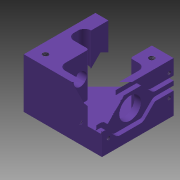
# Autodesk Inventor part: 13_1087_010
Saved by Autodesk Inventor 2014 SP1 (Build 180222100, 222)
## iProperties
Created: 2013-08-07
Part Number: 13_1087_010
Material: Allgemein
Document SubType Name: Modeling
Designer: vogel
Density: 1 g/cm^3
Appearance: Violett
Author: vogel
Autodesk Inventor part; units mm, degrees
note: some values were not read from the file. Chosen so that the rebuilt part matches the saved one: direction of "Bohrung2"; direction of "Bohrung3"; edges of "Rundung6".
ref_plane "YZ Plane" through (0, 0, 0) normal (1, 0, 0) x (0, 1, 0)
ref_plane "XZ Plane" through (0, 0, 0) normal (0, 1, 0) x (-1, 0, 0)
sketch "Skizze1" plane through (0, 0, 0) normal (0, 0, 1) x (1, 0, 0)
  line L0 (-25.2, 0) -> (25.2, 0) projected
  line L1 (0, -25.2) -> (0, 25.2) projected
  line L2 (-18, 18) -> (18, 18)
  line L3 (18, 18) -> (18, -18)
  line L4 (18, -18) -> (-18, -18)
  line L5 (-18, -18) -> (-18, 18)
  point P0 (0, 0)
  dimension "d0" = 36
  dimension "d1" = 36
  constraints: 8 end point, 2 parallel, 1 horizontal, 1 perpendicular, 2 other
  measures "d0" distance of L2.start L2.end
  measures "d1" distance of L4.end L2.start
extrude "Extrusion1" add sketch "Skizze1" along normal blind 23
shell "Hülle1" thickness 3 removed faces 1 at (6, -6, 23)
sketch "Skizze2" plane through (18, -18, 0) normal (1, 0, 0) x (0, 0, -1)
  line L0 (0, 36) -> (0, 0) projected
  line L1 (0, 36) -> (-23, 36) projected
  line L2 (0, 0) -> (-23, 0) projected
  line L3 (-13, 36) -> (-13, 0)
  line L4 (-3, 33) -> (-23, 33) projected
  point P0 (0, 18)
  point P1 (-13, 13)
  dimension "d5" = 13
  dimension "d30" = 20
  constraints: 3 point on line, 2 end point, 1 perpendicular
  measures "d5" distance between parallel lines of L3 L0
  measures "d30" distance from line of point (-13, 13) L4
sketch "Skizze3" plane through (-18, 18, 0) normal (0, 1, 0) x (1, 0, 0)
  line L0 (0, 0) -> (36, 0) projected
  line L1 (33, -3) -> (33, -23) projected
  line L2 (3, -3) -> (33, -3) projected
  line L3 (50, -7) -> (50, -17) projected
  point P0 (18, 0)
  point P1 (13, -13)
  dimension "d13" = 13
  dimension "d14" = 20
  measures "d13" distance from line of point (13, -13) L0
  measures "d14" distance from line of point (13, -13) L1
hole "Bohrung2" at (-5, 18, 13) direction (0, -1, 0) diameter 10 end up to surface
hole "Bohrung3" at (18, -5, 13) direction (-1, 0, 0) diameter 10 end up to surface
sketch "Skizze4" plane through (-15, 15, 3) normal (0, 0, 1) x (1, 0, 0)
  line L0 (0, -30) -> (0, 0) projected
  line L1 (30, -30) -> (0, -30) projected
  line L2 (0, -16) -> (10, -16)
  line L3 (10, -16) -> (10, -30)
  line L4 (10, -30) -> (0, -30)
  line L5 (0, -30) -> (0, -16)
  line L6 (30, 0) -> (23, 0)
  line L7 (23, 0) -> (23, -10)
  line L8 (23, -10) -> (30, -10)
  line L9 (30, -10) -> (30, 0)
  line L10 (0, 0) -> (30, 0) projected
  line L11 (3, 0) -> (0, 0)
  line L12 (0, 0) -> (0, -10)
  line L13 (0, -10) -> (3, -10)
  line L14 (3, -10) -> (3, 0)
  point P0 (15, -15)
  dimension "d31" = 14
  dimension "d32" = 10
  dimension "d40" = 10
  dimension "d41" = 7
  dimension "d46" = 3
  constraints: 24 end point, 6 parallel, 4 point on line, 3 horizontal, 3 perpendicular, 1 collinear
  measures "d31" distance of L4.end L2.start
  measures "d32" distance of L2.start L2.end
  measures "d40" distance between parallel lines of L6 L8
  measures "d41" distance of L7.end L8.end
  measures "d46" distance between parallel lines of L14 L12
extrude "Extrusion2" add sketch "Skizze4" along normal up to surface (20 mm away)
sketch "Skizze8" plane through (-15, 5, 3) normal (0, -1, 0) x (1, 0, 0)
  line L0 (3, 20) -> (0, 20) projected
  line L1 (0, 0) -> (0, 20) projected
  line L2 (3, 0) -> (0, 0) projected
  line L3 (3, 0) -> (3, 20) projected
  point P0 (15, -3)
extrude "Extrusion5" cut sketch "Skizze8" against normal blind 2
fillet "Rundung5" radius 1 2 edges at (-5, -1, 13) (8, 5, 13)
fillet "Rundung6" radius 3 5 edges at (-15, 7, 13) (-15, -1, 13) (-5, -15, 13) (15, -15, 13) (15, 5, 13)
sketch "Skizze9" plane through (18, -18, 0) normal (1, 0, 0) x (0, 0, -1)
  circle A0 centre (-13, 13) radius 5 projected
  point P0 (0, 18)
  constraints: 1 coincident
hole "Bohrung4" at (18, -5, 13) direction (-1, 0, 0) diameter 6 depth 27
sketch "Skizze10" plane through (0, 0, 23) normal (0, 0, 1) x (1, 0, 0)
  line L0 (-12, 15) -> (8, 15) projected
  line L1 (18, -18) -> (18, 18) projected
  line L2 (-18, 18) -> (18, 18)
  line L3 (18, 18) -> (18, 15)
  line L4 (18, 15) -> (-18, 15)
  line L5 (-18, 15) -> (-18, 18)
  point P0 (0, 0)
  constraints: 8 end point, 2 parallel, 1 collinear, 1 horizontal, 1 perpendicular, 1 point on line
extrude "Extrusion6" cut sketch "Skizze10" against normal through all
sketch "Skizze11" plane through (0, 0, 23) normal (0, 0, 1) x (1, 0, 0)
  line L0 (-18, -18) -> (18, -18) projected
  line L1 (-18, 15) -> (-18, -18) projected
  line L2 (18, 15) -> (-18, 15) projected
  line L3 (18, -18) -> (18, 15) projected
  circle A0 centre (-13, -13) radius 1.7 projected
  circle A1 centre (13, 10) radius 1.7 projected
  circle A2 centre (-13, -13) radius 1.7 projected
  point P0 (0, 0)
  point P1 (-13, -13)
  point P2 (13, 10)
hole "Bohrung5" at (-13, -13, 23) at (13, 10, 23) direction (0, 0, -1) diameter 2.459 depth 8 tip angle 118 thread size "M3x0.5" class "6H" standard "ISO Metric profile"
hole "Bohrung6" at (-5, -5, 13) direction (-1, 0, 0) diameter 4 depth 6 tip angle 118
sketch "Skizze12" plane through (-18, -18, 0) normal (0, -1, 0) x (1, 0, 0)
  line L0 (36, 0) -> (0, 0) projected
  line L1 (36, 0) -> (36, 23) projected
  line L2 (36, 9) -> (29.5, 9)
  line L3 (29.5, 9) -> (29.5, 17)
  line L4 (29.5, 17) -> (36, 17)
  line L5 (36, 17) -> (36, 9)
  circle A0 centre (22, 7) radius 2.2 projected
  circle A1 centre (22, 19) radius 2.2 projected
  circle A2 centre (4, 13) radius 2.2 projected
  circle A3 centre (33, 21) radius 1.2 projected
  circle A4 centre (3, 21) radius 1.2 projected
  circle A5 centre (3, 5) radius 1.2 projected
  circle A6 centre (33, 5) radius 1.2 projected
  circle A7 centre (8.5, 13) radius 0.9 projected
  circle A8 centre (17.5, 13) radius 0.9 projected
  circle A9 centre (13, 13) radius 3 projected
  line L6 (0, 0) -> (0, 26) projected
  line L7 (0, 0) -> (36, 0) projected
  line L8 (36, 0) -> (36, 26) projected
  line L9 (0, 26) -> (36, 26) projected
  point P0 (18, 0)
  dimension "d79" = 9
  dimension "d80" = 8
  dimension "d81" = 6.5
  dimension "d94" = 9
  constraints: 8 end point, 2 parallel, 1 horizontal, 1 perpendicular, 1 point on line
  measures "d79" distance between parallel lines of L2 L0
  measures "d80" distance of L2.end L3.end
  measures "d81" distance between parallel lines of L3 L1
  measures "d94" distance between parallel lines of L9 L4
extrude "Extrusion7" add sketch "Skizze12" along normal blind 8 contours L2 L3 L4 L1
sketch "Skizze14" plane through (18, -18, 0) normal (1, 0, 0) x (0, 0, -1)
  line L0 (0, 33) -> (-23, 33) projected
  line L1 (-23, 0) -> (-23, 33) projected
  line L2 (-9, -8) -> (-17, -8) projected
  line L3 (0, 0) -> (-9, 0) projected
  line L4 (0, 33) -> (0, 0) projected
  circle A0 centre (-13, 13) radius 5 projected
  line L5 (-11, -8) -> (-11, 1.1716)
  line L6 (-10.4142, 2.5858) -> (-6.0858, 6.9142)
  line L7 (-5.5, 8.3284) -> (-5.5, 17.6716)
  line L8 (-15, -8) -> (-15, 1.1716)
  line L9 (-15.5858, 2.5858) -> (-19.9142, 6.9142)
  line L10 (-20.5, 8.3284) -> (-20.5, 23.6063)
  line L11 (-13, 13) -> (-13, 24.4674)
  line L12 (-13, 24.4674) -> (-13, 13)
  line L13 (-10.2295, 13) -> (-13, 13)
  line L14 (-13, 13) -> (-13, -8)
  arc A1 (-10.4142, 2.5858) -> (-11, 1.1716) centre (-9, 1.1716) ccw
  arc A2 (-15, 1.1716) -> (-15.5858, 2.5858) centre (-17, 1.1716) ccw
  arc A3 (-20.5, 8.3284) -> (-19.9142, 6.9142) centre (-18.5, 8.3284) ccw
  arc A4 (-6.0858, 6.9142) -> (-5.5, 8.3284) centre (-7.5, 8.3284) ccw
  line L15 (-9, 0) -> (-9, -8) projected
  line L16 (-6.0858, 19.0858) -> (-10.4142, 23.4142)
  line L17 (-11, 24.8284) -> (-11, 33)
  arc A5 (-5.5, 17.6716) -> (-6.0858, 19.0858) centre (-7.5, 17.6716) ccw
  arc A6 (-11, 24.8284) -> (-10.4142, 23.4142) centre (-9, 24.8284) ccw
  point P0 (-17, 0)
  point P1 (0, 18)
  point P2 (-11, 2)
  point P3 (-5.5, 18.5)
  point P4 (-11, 24)
  dimension "d87" = 45
  dimension "d89" = 9
  dimension "d90" = 6
  dimension "d91" = 13
  dimension "d92" = 10
  dimension "d93" = 8
  dimension "d96" = 4
  dimension "d97" = 15
  dimension "d98" = 2
  dimension "d99" = 2
  dimension "d108" = 45
  dimension "d109" = 24
  dimension "d110" = 2
  dimension "d139" = 9
  constraints: 24 end point, 12 point on circle, 12 tangent, 9 point on line, 6 centre point, 6 parallel, 4 equal radius, 2 collinear, 2 perpendicular, 1 midpoint, 3 other
  measures "d87" angle of L3 L6
  measures "d89" distance of L3.start L3.end
  measures "d90" distance of point (-17, 0) L1.start
  measures "d91" distance between parallel lines of L4 L11
  measures "d92" distance between parallel lines of L1 L11
  measures "d93" distance of L2.start L2.end
  measures "d96" distance of L8.start L5.start
  measures "d97" distance between parallel lines of L7 L10
  measures "d98" distance from line of point (-11, 2) L3
  measures "d99" radius of A1
  measures "d108" angle of L16 L0
  measures "d109" distance from line of point (-11, 24) L3
  measures "d110" radius of A5
  measures "d139" distance from line of point (-11, 24) L0
sketch "Skizze15" plane through (-18, -26, 0) normal (0, -1, 0) x (1, 0, 0)
  line L0 (36, 9) -> (36, 17) projected
  line L1 (36, 10) -> (34, 10)
  line L2 (34, 10) -> (34, 12)
  line L3 (34, 12) -> (36, 12)
  line L4 (36, 12) -> (36, 10)
  line L5 (36, 14) -> (34, 14)
  line L6 (34, 14) -> (34, 16)
  line L7 (34, 16) -> (36, 16)
  line L8 (36, 16) -> (36, 14)
  line L9 (36, 15) -> (34, 15)
  line L10 (36, 11) -> (34.6551, 11)
  point P0 (18, 0)
  point P1 (36, 15)
  point P2 (36, 11)
  dimension "d100" = 2
  dimension "d101" = 2
  dimension "d102" = 2
  dimension "d103" = 2
  constraints: 20 end point, 4 parallel, 4 perpendicular, 2 horizontal, 1 collinear, 1 midpoint, 1 point on line, 2 other
  measures "d100" distance of L5.end L6.end
  measures "d101" distance between parallel lines of L6 L0
  measures "d102" distance between parallel lines of L3 L1
  measures "d103" distance between parallel lines of L2 L0
sweep "Sweeping1" cut profiles "Skizze15" path "Skizze14" path curves L5 A1 L6 A4 L7 A5 L16 A6 L17 contours L1 L2 L3 L0
ref_plane "Arbeitsebene1" through (0, 0, 13) normal (0, 0, -1) x (-1, 0, 0)
mirror "Spiegeln2" about plane through (0, 0, 13) normal (0, 0, -1) of "Sweeping1"
sketch "Skizze18" plane through (8, 15, 23) normal (0, 1, 0) x (1, 0, 0)
  circle A0 centre (-23, 18) radius 1.2 projected
  circle A1 centre (-23, 2) radius 1.2 projected
  circle A2 centre (7, 18) radius 1.2 projected
  circle A3 centre (7, 2) radius 1.2 projected
  point P0 (-8, 23)
  constraints: 4 coincident
hole "Bohrung8" at (-15, 15, 5) at (15, 15, 5) at (15, 15, 21) at (-15, 15, 21) direction (0, -1, 0) diameter 1.567 depth 6 tip angle 118 thread size "M2x0.4" class "6H" standard "ISO Metric profile"
sketch "Skizze17" plane through (18, -18, 23) normal (1, 0, 0) x (0, 0, -1)
  line L0 (7, 24.8284) -> (7, 33) projected
  line L1 (7, 33) -> (0, 33) projected
  line L2 (0, 0) -> (0, 33) projected
  line L3 (6, 0) -> (0, 0) projected
  line L4 (6, 0) -> (6, -8) projected
  line L5 (7, -8) -> (6, -8) projected
  line L6 (7, -8) -> (7, 1.1716) projected
  arc A0 (7, 1.1716) -> (6.7071, 1.8787) centre (6, 1.1716) ccw projected
  line L7 (6.7071, 1.8787) -> (2.3787, 6.2071) projected
  arc A1 (1.5, 8.3284) -> (2.3787, 6.2071) centre (4.5, 8.3284) ccw projected
  line L8 (1.5, 8.3284) -> (1.5, 17.6716) projected
  arc A2 (2.3787, 19.7929) -> (1.5, 17.6716) centre (4.5, 17.6716) ccw projected
  line L9 (2.3787, 19.7929) -> (6.7071, 24.1213) projected
  arc A3 (6.7071, 24.1213) -> (7, 24.8284) centre (6, 24.8284) ccw projected
  circle A4 centre (5, 31) radius 1.2 projected
  line L10 (13, 33) -> (13, 24.8284) projected
  arc A5 (13, 24.8284) -> (13.2929, 24.1213) centre (14, 24.8284) ccw projected
  line L11 (13.2929, 24.1213) -> (17.6213, 19.7929) projected
  arc A6 (18.5, 17.6716) -> (17.6213, 19.7929) centre (15.5, 17.6716) ccw projected
  line L12 (18.5, 17.6716) -> (18.5, 8.3284) projected
  arc A7 (17.6213, 6.2071) -> (18.5, 8.3284) centre (15.5, 8.3284) ccw projected
  line L13 (17.6213, 6.2071) -> (13.2929, 1.8787) projected
  arc A8 (13.2929, 1.8787) -> (13, 1.1716) centre (14, 1.1716) ccw projected
  line L14 (13, 1.1716) -> (13, -8) projected
  line L15 (14, -8) -> (13, -8) projected
  line L16 (14, 0) -> (14, -8) projected
  line L17 (23, 0) -> (14, 0) projected
  line L18 (23, 33) -> (23, 0) projected
  line L19 (23, 33) -> (13, 33) projected
  circle A9 centre (15, 31) radius 1.2 projected
  circle A10 centre (17, 3) radius 1.2 projected
  circle A11 centre (3, 3) radius 1.2 projected
  point P0 (23, 18)
  constraints: 4 coincident
hole "Bohrung9" at (18, 13, 18) at (18, 13, 8) at (18, -15, 6) at (18, -15, 20) direction (-1, 0, 0) diameter 1.567 depth 6 tip angle 118 thread size "M2x0.4" class "6H" standard "ISO Metric profile"
sketch "Skizze19" plane through (11.5, -18, 9) normal (-1, 0, 0) x (0, 0, 1)
  circle A0 centre (4, -4) radius 1.7 projected
  point P0 (-9, 18)
  constraints: 1 coincident
hole "Bohrung10" at (11.5, -22, 13) direction (1, 0, 0) diameter 2.459 depth 5 tip angle 118 thread size "M3x0.5" class "6H" standard "ISO Metric profile"
